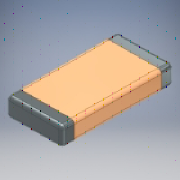
# Autodesk Inventor part: 1206_Cap
Saved by Autodesk Inventor 2017 SP1 (Build 210196100, 196)
## iProperties
Created: 2016-08-27
Part Number: 1206_Cap
Material: Lead
Document SubType Name: Modeling
Designer: jwrjc
Language: en-US
Size Designation: 1206_Cap
Categories: <MemberInstance><Categories><Category DisplayName="Electrical" InternalName="690189fb-5335-48bc-ba8f-fa4ddabb13bb" Mnemonic="IDF"><Category DisplayName="Components" InternalName="eab5d76b-1861-4102-82a0-277eae840d4a" Mnemonic="COMPONENTS"><Category DisplayName="Electrical" InternalName="e935d458-c05c-4f25-8523-65af19dfc39b" Mnemonic="ELECTRICAL"><Category DisplayName="Capacitors" InternalName="2c04a40c-fbe6-4b69-b807-de3546ef4c59" Mnemonic="CAPACITORS"/></Category></Category></Category><Category DisplayName="DataType" InternalName="23b78d0f-2648-40c6-8793-ca6db495c9e8" Mnemonic="DATATYPE"><CategoryParameter DisplayName="DisplayName" InternalName="05415f3d-3907-474b-a020-eb9d644f4cf3" Mnemonic="DISPLAYNAME"/><CategoryParameter DisplayName="Standard" InternalName="0c0a119c-1e12-4c84-803f-101930972f5e" Mnemonic="STANDARD"/><CategoryParameter DisplayName="Description" InternalName="13903e3d-64b1-4950-80da-f627842ea37f" Mnemonic="DESCRIPTION"/><CategoryParameter DisplayName="Designation" InternalName="2675968c-4ce5-49e0-a4f5-552d29089031" Mnemonic="DESIGNATION"/><CategoryParameter DisplayName="Default Row" InternalName="2af9ec52-faaa-4026-b378-f9fa4afca842" Mnemonic="DEFAULTROW"/><CategoryParameter DisplayName="Folder Name" InternalName="3f06958e-8713-4116-9be7-ed6184ecc97b" Mnemonic="FOLDERNAME"/><CategoryParameter DisplayName="Revision Guid" InternalName="45a75005-10b1-4dfc-8d6d-dfe629f0b93c" Mnemonic="REVISIONGUID"/><CategoryParameter DisplayName="FileName" InternalName="8b46a4cc-9585-4fed-90c3-899f57e09a73" Mnemonic="FILENAME"/><CategoryParameter DisplayName="StdsOrg" InternalName="8f5914e1-4693-403f-8ab5-d37768198c9d" Mnemonic="STDSORG"/><CategoryParameter DisplayName="Family Version" InternalName="914462f6-6e19-4b14-ba84-155b9680b1d0" Mnemonic="FAMILYREVISION"/><CategoryParameter DisplayName="Standard Revision" InternalName="91d5a463-65c2-4fde-b823-3b7fea5e8e17" Mnemonic="STANDARDREVISION"/><CategoryParameter DisplayName="Member Revision" InternalName="a65d44b9-392f-4f4f-857b-e4b3d54996fe" Mnemonic="MEMBERREVISION"/><CategoryParameter DisplayName="ClipFormat" InternalName="bc51e27b-3422-4e78-93ef-cec197ddf230" Mnemonic="CLIPFORMAT"/><CategoryParameter DisplayName="Manufacturer" InternalName="cd6c7a72-a28a-4e50-99a9-2c7f4e13e5ad" Mnemonic="MANUFACTURER"/><CategoryParameter DisplayName="InternalName" InternalName="cf1d0246-76d9-4b4a-8305-fa0409afb5c1" Mnemonic="INTERNALNAME"/><CategoryParameter DisplayName="IsMetric" InternalName="e2385c5b-1ea4-4823-96a8-8de651266ec3" Mnemonic="ISMETRIC"/><Category DisplayName="Part" InternalName="c0e0b642-3bcb-4cc8-9e80-f96d35c4afa4" Mnemonic="PART"><CategoryParameter DisplayName="Part Number" InternalName="016b6077-bfbe-49bd-92c9-d8d59c39c941" Mnemonic="PARTNUMBER"/><CategoryParameter DisplayName="Stock Number" InternalName="4dba7c1c-e26c-444e-836c-b08b433409a8" Mnemonic="STOCKNUMBER"/><CategoryParameter DisplayName="Material Key" InternalName="5c9a8adb-dd2b-4535-b97f-0a94a95fe41f" Mnemonic="MATERIALKEY"/><CategoryParameter DisplayName="Material" InternalName="818a152a-d3c3-49ca-80ee-df7d91421b8e" Mnemonic="MATERIAL"/></Category></Category></Categories><FamilyTemplate Id="1206_Cap"><FamilyTemplateParameters><FamilyTemplateParameter ObjectType="kPartComponentDefinitionObject" ValueType="xs:string" Id="11" SubObjectId="Material"/><FamilyTemplateParameter ObjectType="kPropertyObject" ValueType="xs:string" Id="15" ObjectReferenceKey="{32853F0F-3444-11d1-9E93-0060B03C1CA6}" SubObjectId="5"/><FamilyTemplateParameter ObjectType="kPropertyObject" ValueType="xs:string" Id="16" ObjectReferenceKey="{32853F0F-3444-11d1-9E93-0060B03C1CA6}" SubObjectId="52"/></FamilyTemplateParameters></FamilyTemplate><CategoryParameterMap><ParamToTemplateMap><ParamToTemplate CategoryParameter="//CategoryParameter[@InternalName='cf1d0246-76d9-4b4a-8305-fa0409afb5c1']" ConstantValue="a1b847e4-773b-4ad0-9d2e-54362debdea1"/><ParamToTemplate CategoryParameter="//CategoryParameter[@InternalName='45a75005-10b1-4dfc-8d6d-dfe629f0b93c']" ConstantValue="50045446-f274-43cc-ada6-68913090cdfb"/><ParamToTemplate CategoryParameter="//CategoryParameter[@InternalName='3f06958e-8713-4116-9be7-ed6184ecc97b']" ConstantValue="1206_SMD"/><ParamToTemplate CategoryParameter="//CategoryParameter[@InternalName='8f5914e1-4693-403f-8ab5-d37768198c9d']" TemplateParameter="5"/><ParamToTemplate CategoryParameter="//CategoryParameter[@InternalName='0c0a119c-1e12-4c84-803f-101930972f5e']" TemplateParameter="6"/><ParamToTemplate CategoryParameter="//CategoryParameter[@InternalName='91d5a463-65c2-4fde-b823-3b7fea5e8e17']" TemplateParameter="7"/><ParamToTemplate CategoryParameter="//CategoryParameter[@InternalName='cd6c7a72-a28a-4e50-99a9-2c7f4e13e5ad']" TemplateParameter="8"/><ParamToTemplate CategoryParameter="//CategoryParameter[@InternalName='13903e3d-64b1-4950-80da-f627842ea37f']" TemplateParameter="10"/><ParamToTemplate CategoryParameter="//CategoryParameter[@InternalName='05415f3d-3907-474b-a020-eb9d644f4cf3']" ConstantValue="1206_SMD"/><ParamToTemplate CategoryParameter="//CategoryParameter[@InternalName='914462f6-6e19-4b14-ba84-155b9680b1d0']" ConstantValue="11"/><ParamToTemplate CategoryParameter="//CategoryParameter[@InternalName='bc51e27b-3422-4e78-93ef-cec197ddf230']" ConstantValue="CF_INVENTOR.STDPARTS"/><ParamToTemplate CategoryParameter="//CategoryParameter[@InternalName='e2385c5b-1ea4-4823-96a8-8de651266ec3']" ConstantValue="true"/><ParamToTemplate CategoryParameter="//CategoryParameter[@InternalName='2af9ec52-faaa-4026-b378-f9fa4afca842']" ConstantValue="1"/><ParamToTemplate CategoryParameter="//CategoryParameter[@InternalName='8b46a4cc-9585-4fed-90c3-899f57e09a73']" ConstantValue="1206_Cap"/><ParamToTemplate CategoryParameter="//CategoryParameter[@InternalName='a65d44b9-392f-4f4f-857b-e4b3d54996fe']" ConstantValue="094538be-b72c-443c-95dc-e7385b61e7b9"/><ParamToTemplate CategoryParameter="//CategoryParameter[@InternalName='a65d44b9-392f-4f4f-857b-e4b3d54996fe']" ConstantValue="094538be-b72c-443c-95dc-e7385b61e7b9"/><ParamToTemplate CategoryParameter="//CategoryParameter[@InternalName='2675968c-4ce5-49e0-a4f5-552d29089031']" TemplateParameter="16"/><ParamToTemplate CategoryParameter="//CategoryParameter[@InternalName='818a152a-d3c3-49ca-80ee-df7d91421b8e']" TemplateParameter="11"/><ParamToTemplate CategoryParameter="//CategoryParameter[@InternalName='016b6077-bfbe-49bd-92c9-d8d59c39c941']" TemplateParameter="15"/></ParamToTemplateMap></CategoryParameterMap></MemberInstance>
Density: 11.34 g/cm^3
Appearance: Lead
IsCustomPart: 0
Author: jwrjc
Autodesk Inventor part; units mm, degrees
ref_plane "YZ Plane" through (0, 0, 0) normal (1, 0, 0) x (0, 1, 0)
ref_plane "XZ Plane" through (0, 0, 0) normal (0, 1, 0) x (-1, 0, 0)
ref_plane "XY Plane" through (0, 0, 0) normal (0, 0, 1) x (1, 0, 0)
sketch "Sketch1" plane through (0, 0, 0) normal (0, 0, 1) x (1, 0, 0)
  line L0 (-12.9312, 13.1313) -> (-11.3312, 13.1313)
  line L1 (-11.3312, 13.1313) -> (-11.3312, 10.6313)
  line L2 (-11.3312, 10.6313) -> (-12.9312, 10.6313)
  line L3 (-12.9312, 10.6313) -> (-12.9312, 13.1313)
  line L4 (-12.9312, 10.6313) -> (-11.3312, 10.6313)
  line L5 (-11.3312, 10.6313) -> (-11.3312, 10.2813)
  line L6 (-11.3312, 10.2813) -> (-12.9312, 10.2813)
  line L7 (-12.9312, 10.2813) -> (-12.9312, 10.6313)
  line L8 (-12.9312, 13.4813) -> (-11.3312, 13.4813)
  line L9 (-11.3312, 13.4813) -> (-11.3312, 13.1313)
  line L10 (-11.3312, 13.1313) -> (-12.9312, 13.1313)
  line L11 (-12.9312, 13.1313) -> (-12.9312, 13.4813)
  point P0 (0, 0)
  dimension "d0" = 1.6
  dimension "d1" = 2.5
  dimension "d2" = 3.2
  dimension "d3" = 0.35
  constraints: 24 end point, 6 parallel, 4 point on line, 3 horizontal, 3 perpendicular, 2 collinear
  measures "d0" distance of L1.end L2.end
  measures "d1" distance of L0.end L1.end
  measures "d2" distance between parallel lines of L6 L8
  measures "d3" distance between parallel lines of L2 L6
extrude "Extrusion1" add sketch "Sketch1" along normal blind 0.55 contours L0 L1 L2 L3
extrude "Extrusion2" add sketch "Sketch1" along normal blind 0.55 separate body contours L11 L8 L9 L0 | L2 L5 L6 L7
fillet "Fillet1" radius 0.1 20 edges at (-12.9312, 11.8813, 0.55) (-11.3312, 11.8813, 0.55) (-11.3312, 11.8813, 0) (-12.9312, 11.8813, 0) (-12.9312, 10.4563, 0.55) (-12.9312, 13.3063, 0.55) (-12.1312, 13.4813, 0.55) (-11.3312, 13.3063, 0.55) (-11.3312, 10.4563, 0.55) (-12.1312, 10.2813, 0.55) (-11.3312, 10.2813, 0.275) (-12.9312, 10.2813, 0.275) (-12.1312, 10.2813, 0) (-11.3312, 10.4563, 0) (-11.3312, 13.3063, 0) (-11.3312, 13.4813, 0.275) (-12.9312, 10.4563, 0) (-12.9312, 13.3063, 0) (-12.9312, 13.4813, 0.275) (-12.1312, 13.4813, 0)
body "Solid1"
body "Solid2"
